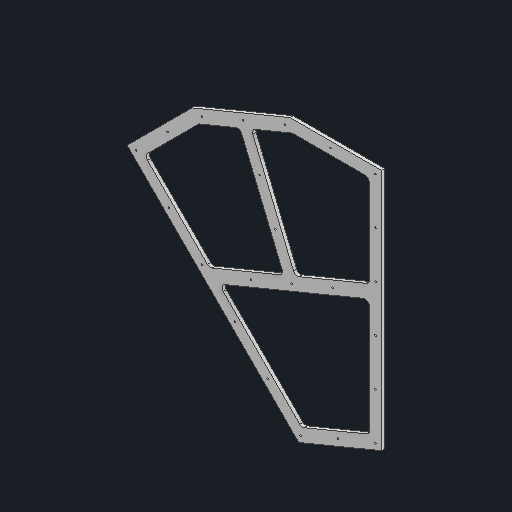
# Autodesk Inventor part: DMF 01 56 Крепление сетки к кассете v2.1
Saved by Autodesk Inventor 2026.2 (Build 302298010, 298A)
## iProperties
Created: 2024-05-05
Part Number: DMF 01 56 Крепление сетки к кассете v2.1
Material: Generic
Document SubType Name: Modeling
Designer: pokla
Density: 1 g/cm^3
Appearance: Default
Author: pokla
Autodesk Inventor part; units mm, degrees
ref_plane "YZ Plane" through (0, 0, 0) normal (1, 0, 0) x (0, 1, 0)
ref_plane "XZ Plane" through (0, 0, 0) normal (0, 1, 0) x (-1, 0, 0)
ref_plane "XY Plane" through (0, 0, 0) normal (0, 0, 1) x (1, 0, 0)
sketch "Sketch1" plane through (0, 0, 0) normal (0, 0, 1) x (1, 0, 0)
  line L0 (0, 286.8339) -> (202.8222, 202.8222) construction
  line L1 (202.8222, 202.8222) -> (286.8339, 0) construction
  line L2 (286.8339, 0) -> (202.8222, -202.8222) construction
  line L3 (202.8222, -202.8222) -> (0, -286.8339) construction
  line L4 (0, -286.8339) -> (-202.8222, -202.8222) construction
  line L5 (-202.8222, -202.8222) -> (-286.8339, 0) construction
  line L6 (-286.8339, 0) -> (-202.8222, 202.8222) construction
  line L7 (-202.8222, 202.8222) -> (0, 286.8339)
  line L8 (-202.8222, 202.8222) -> (0, 286.8339)
  line L9 (-464.5194, 781.7427) -> (-224.3107, 881.2404)
  line L10 (-101.4111, 244.8281) -> (-344.4151, 831.4916) construction
  line L11 (-224.3107, 881.2404) -> (0, 881.2404)
  line L12 (0, 881.2404) -> (0, 286.8339)
  line L13 (-464.5194, 781.7427) -> (-623.1311, 623.1311)
  line L14 (-623.1311, 623.1311) -> (-202.8222, 202.8222)
  point P0 (0, 0)
  point P1 (0, 0)
  dimension "d0" = 530
  dimension "d2" = 260
  dimension "d3" = 635
  constraints: 30 end point, 2 midpoint, 1 coincident, 1 horizontal, 1 parallel, 1 perpendicular, 1 symmetric about line, 1 vertical, 1 vertical alignment, 17 other
  measures "d0" distance between parallel lines of L5 L1
  measures "d2" distance of L9.start L9.end
  measures "d3" distance of L10.end L10.start
extrude "Extrusion1" add sketch "Sketch1" along normal mid plane 8
sketch "Sketch2" plane through (0, 0, 4) normal (0, 0, 1) x (1, 0, 0)
  line L0 (-224.3107, 881.2404) -> (-464.5194, 781.7427) projected
  line L1 (-464.5194, 781.7427) -> (-623.1311, 623.1311) projected
  line L2 (-239.6414, 539.3487) -> (-421.5665, 463.9929)
  line L3 (-202.8222, 202.8222) -> (0, 286.8339) projected
  line L4 (-101.4111, 244.8281) -> (-344.4151, 831.4916) construction
  line L5 (-623.1311, 623.1311) -> (-202.8222, 202.8222) projected
  line L6 (-421.5665, 463.9929) -> (-580.7047, 623.1311)
  line L7 (-580.7047, 623.1311) -> (-447.5258, 756.31)
  line L8 (-447.5258, 756.31) -> (-346.7928, 798.0349)
  line L9 (-239.6414, 539.3487) -> (-346.7928, 798.0349)
  line L10 (-211.925, 550.8292) -> (-30, 626.185)
  line L11 (-30, 626.185) -> (-30, 851.2404)
  line L12 (-30, 851.2404) -> (-218.3434, 851.2404)
  line L13 (-218.3434, 851.2404) -> (-319.0764, 809.5154)
  line L14 (-211.925, 550.8292) -> (-319.0764, 809.5154)
  line L15 (0, 286.8339) -> (0, 881.2404) projected
  line L16 (-421.5665, 463.9929) -> (-30, 626.185) construction
  line L17 (-398.6054, 441.0319) -> (-30, 593.7132)
  line L18 (-195.7832, 238.2096) -> (-30, 306.8793)
  line L19 (-30, 306.8793) -> (-30, 593.7132)
  line L20 (-195.7832, 238.2096) -> (-398.6054, 441.0319)
  point P0 (0, 0)
  dimension "d11" = 30
  dimension "d12" = 280
  dimension "d13" = 30
  dimension "d14" = 30
  dimension "d15" = 15
  dimension "d21" = 30
  dimension "d22" = 30
  dimension "d23" = 30
  dimension "d24" = 30
  constraints: 32 end point, 5 parallel, 5 symmetric about line, 2 midpoint, 1 collinear
  measures "d11" distance between parallel lines of L5 L6
  measures "d12" distance between parallel lines of L8 L2
  measures "d13" distance between parallel lines of L0 L8
  measures "d14" distance between parallel lines of L1 L7
  measures "d15" distance between parallel lines of L9 L4
  measures "d21" distance between parallel lines of L16 L17
  measures "d22" distance between parallel lines of L5 L20
  measures "d23" distance between parallel lines of L19 L15
  measures "d24" distance between parallel lines of L18 L3
extrude "Extrusion2" cut sketch "Sketch2" against normal up to surface (8 mm away)
fillet "Fillet1" radius 10 12 edges at (-580.7047, 623.1311, 0) (-346.7928, 798.0349, 0) (-239.6414, 539.3487, 0) (-421.5665, 463.9929, 0) (-319.0764, 809.5154, 0) (-30, 851.2404, 0) (-30, 626.185, 0) (-211.925, 550.8292, 0) (-398.6054, 441.0319, 0) (-30, 593.7132, 0) (-30, 306.8793, 0) (-195.7832, 238.2096, 0)
sketch "Sketch5" plane through (0, 0, 4) normal (0, 0, 1) x (1, 0, 0)
  line L0 (-224.3107, 881.2404) -> (-464.5194, 781.7427) projected
  line L1 (0, 881.2404) -> (-224.3107, 881.2404) projected
  line L2 (-464.5194, 781.7427) -> (-623.1311, 623.1311) projected
  line L3 (-623.1311, 623.1311) -> (-202.8222, 202.8222) projected
  line L4 (-202.8222, 202.8222) -> (0, 286.8339) projected
  line L5 (0, 286.8339) -> (0, 881.2404) projected
  line L6 (-15, 866.2404) -> (-221.3271, 866.2404) construction
  line L7 (-221.3271, 866.2404) -> (-456.0226, 769.0263) construction
  line L8 (-456.0226, 769.0263) -> (-601.9179, 623.1311) construction
  line L9 (-601.9179, 623.1311) -> (-199.3027, 220.5159) construction
  line L10 (-199.3027, 220.5159) -> (-15, 296.8566) construction
  line L11 (-15, 296.8566) -> (-15, 866.2404) construction
  line L12 (-384.7786, 446.7591) -> (-43.8268, 587.986) projected
  line L13 (-215.7519, 560.068) -> (-315.2496, 800.2766) projected
  line L14 (-425.0859, 446.2992) -> (-15, 616.1623) construction
  line L15 (-220.043, 531.2307) -> (-338.6748, 817.6334) construction
  circle A0 centre (-338.6748, 817.6334) radius 2
  circle A1 centre (-220.043, 531.2307) radius 2
  circle A2 centre (-299.1322, 722.1689) radius 2
  circle A3 centre (-259.5895, 626.7044) radius 2
  circle A4 centre (-601.9179, 623.1311) radius 2
  circle A5 centre (-521.1258, 542.339) radius 2
  circle A6 centre (-440.3338, 461.547) radius 2
  circle A7 centre (-359.5418, 380.755) radius 2
  circle A8 centre (-278.7497, 299.9629) radius 2
  circle A9 centre (-197.9577, 219.1709) radius 2
  circle A10 centre (-320.2839, 489.7096) radius 2
  circle A11 centre (-107.1514, 258.6863) radius 2
  circle A12 centre (-524.1361, 700.9128) radius 2
  circle A13 centre (-440.3016, 775.5382) radius 2
  circle A14 centre (-15, 866.2404) radius 2
  circle A15 centre (-15, 751.9832) radius 2
  circle A16 centre (-15, 637.726) radius 2
  circle A17 centre (-15, 523.4688) radius 2
  circle A18 centre (-15, 409.2116) radius 2
  circle A19 centre (-15, 294.9544) radius 2
  circle A20 centre (-119.802, 572.7519) radius 2
  circle A21 centre (-125, 866.2404) radius 2
  circle A22 centre (-237.0481, 859.7286) radius 2
  point P0 (0, 0)
  dimension "d32" = 15
  dimension "d33" = 15
  dimension "d34" = 15
  dimension "d35" = 4
  dimension "d37" = 103.33
  dimension "d38" = 103.33
  dimension "d43" = 114.2572
  dimension "d49" = 108.5
  dimension "d50" = 110
  dimension "d51" = 110
  constraints: 23 centre point, 16 end point, 9 symmetric about line, 8 equal radius, 7 point on line, 3 coincident, 3 midpoint, 2 parallel, 25 other
  measures "d32" distance between parallel lines of L5 L11
  measures "d33" distance between parallel lines of L12 L14
  measures "d34" distance between parallel lines of L13 L15
  measures "d35" diameter of A0
  measures "d37" distance of A2.centre A0.centre
  measures "d38" distance of A3.centre A2.centre
  measures "d43" distance of A4.centre A5.centre
  measures "d49" distance of A1.centre A10.centre
  measures "d50" distance of A12.centre A4.centre
  measures "d51" distance of A13.centre A0.centre
extrude "Extrusion4" cut sketch "Sketch5" against normal up to surface (8 mm away) contours A0 | A1 | A2 | A3 | A4 | A5 | A6 | A7 | A8 | A9 | A10 | A11 | A12 | A13 | A14 | A15 | A16 | A17 | A18 | A19 | A20 | A21 | A22
equation "\"d0\" = Барабан_размер_по_плоскостям"
equation "\"d2\" = Кассета_длина_грани"
equation "\"d3\" = Кассета_высота"
equation "\"d11\" = d13"
equation "\"d14\" = d13"
equation "\"d15\" = 0.5 * d13"
equation "\"d21\" = d13"
equation "\"d22\" = d13"
equation "\"d23\" = d13"
equation "\"d24\" = d13"
equation "\"Барабан_размер_по_плоскостям\" = 530"
equation "\"Кассета_длина_грани\" = 260"
equation "\"Кассета_высота\" = 635"
body "Solid1"
